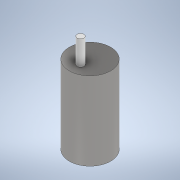
# Autodesk Inventor part: gearmotor
Saved by Autodesk Inventor 2022.2 (Build 262287010, 287A)
## iProperties
Created: 2022-03-26
Part Number: gearmotor
Material: Generic
Document SubType Name: Modeling
Designer: Santiago Larraín
Density: 1 g/cm^3
Appearance: Default
Author: Santiago Larraín
Autodesk Inventor part; units mm, degrees
ref_plane "YZ Plane" through (0, 0, 0) normal (1, 0, 0) x (0, 1, 0)
ref_plane "XZ Plane" through (0, 0, 0) normal (0, 1, 0) x (-1, 0, 0)
ref_plane "XY Plane" through (0, 0, 0) normal (0, 0, 1) x (1, 0, 0)
sketch "Sketch1" plane through (0, 0, 0) normal (0, 1, 0) x (-1, 0, 0)
  circle A0 centre (0, 0) radius 18.5
  dimension "d0" = 37
  constraints: 1 centre point, 1 coincident
  measures "d0" diameter of A0
extrude "Extrusion1" add sketch "Sketch1" along normal blind 70.1
sketch "Sketch2" plane through (0, 70.1, 0) normal (0, 1, 0) x (1, 0, 0)
  circle A0 centre (0, -8.5) radius 6
  circle A1 centre (0, -8.5) radius 3
  point P0 (0, 0)
  dimension "d3" = 12
  dimension "d4" = 6
  constraints: 2 centre point, 1 coincident
  measures "d3" diameter of A0
  measures "d4" diameter of A1
extrude "Extrusion2" add sketch "Sketch2" along normal blind 22 contours A1
body "Solid1"
